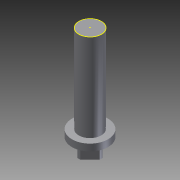
# Autodesk Inventor part: Поз12 Стержень
Saved by Autodesk Inventor 2012 SP2 (Build 160219200, 219)
## iProperties
Created: 2014-04-06
Part Number: Поз12 Стержень
Material: Default
Document SubType Name: Modeling
Designer: N750
Density: 1 g/cm^3
Author: N750
Autodesk Inventor part; units mm, degrees
ref_plane "YZ Plane" through (0, 0, 0) normal (1, 0, 0) x (0, 1, 0)
ref_plane "XZ Plane" through (0, 0, 0) normal (0, 1, 0) x (-1, 0, 0)
ref_plane "XY Plane" through (0, 0, 0) normal (0, 0, 1) x (1, 0, 0)
sketch "Эскиз1" plane through (0, 0, 0) normal (0, 0, 1) x (1, 0, 0)
  circle A0 centre (0, 0) radius 5
  dimension "d0" = 10
  constraints: 1 centre point, 1 coincident
  measures "d0" diameter of A0
extrude "Выдавливание1" add sketch "Эскиз1" along normal blind 6
sketch "Эскиз2" plane through (0, 0, 6) normal (0, 0, 1) x (1, 0, 0)
  circle A0 centre (0, 0) radius 5 projected
  line L0 (0, 5.6569) -> (5.6569, 0)
  line L1 (5.6569, 0) -> (0, -5.6569)
  line L2 (0, -5.6569) -> (-5.6569, 0)
  line L3 (-5.6569, 0) -> (0, 5.6569)
  dimension "d3" = 8
  constraints: 8 end point, 1 coincident, 9 other
  measures "d3" distance of L0.end L1.end
extrude "Выдавливание2" cut sketch "Эскиз2" against normal blind 6 contours A0 L1 L2 L3 L0 | A0 L0 L1 | A0 L3 L0 | L1 L2 A0 | A0 L2 L3 keep common part
sketch "Эскиз3" plane through (0, 0, 6) normal (0, 0, 1) x (1, 0, 0)
  line L0 (-0.7071, -4.9497) -> (-4.9497, -0.7071) projected
  arc A0 (-0.7071, -4.9497) -> (0.7071, -4.9497) centre (0, 0) ccw projected
  line L1 (4.9497, -0.7071) -> (0.7071, -4.9497) projected
  arc A1 (4.9497, -0.7071) -> (4.9497, 0.7071) centre (0, 0) ccw projected
  line L2 (0.7071, 4.9497) -> (4.9497, 0.7071) projected
  arc A2 (0.7071, 4.9497) -> (-0.7071, 4.9497) centre (0, 0) ccw projected
  line L3 (-4.9497, 0.7071) -> (-0.7071, 4.9497) projected
  arc A3 (-4.9497, 0.7071) -> (-4.9497, -0.7071) centre (0, 0) ccw projected
  circle A4 centre (0, 0) radius 8
  dimension "d6" = 16
  constraints: 1 centre point, 1 coincident
  measures "d6" diameter of A4
extrude "Выдавливание3" add sketch "Эскиз3" along normal blind 3
sketch "Эскиз4" plane through (0, 0, 9) normal (0, 0, 1) x (1, 0, 0)
  arc A0 (-4.9497, 0.7071) -> (-4.9497, -0.7071) centre (0, 0) ccw projected
  line L0 (-4.9497, 0.7071) -> (-0.7071, 4.9497) projected
  arc A1 (0.7071, 4.9497) -> (-0.7071, 4.9497) centre (0, 0) ccw projected
  line L1 (0.7071, 4.9497) -> (4.9497, 0.7071) projected
  arc A2 (4.9497, -0.7071) -> (4.9497, 0.7071) centre (0, 0) ccw projected
  line L2 (4.9497, -0.7071) -> (0.7071, -4.9497) projected
  arc A3 (-0.7071, -4.9497) -> (0.7071, -4.9497) centre (0, 0) ccw projected
  line L3 (-0.7071, -4.9497) -> (-4.9497, -0.7071) projected
extrude "Выдавливание4" add sketch "Эскиз4" against normal blind 3
sketch "Эскиз5" plane through (0, 0, 9) normal (0, 0, 1) x (1, 0, 0)
  circle A0 centre (0, 0) radius 8 projected
  circle A1 centre (0, 0) radius 5
  dimension "d11" = 10
  constraints: 1 centre point, 1 coincident
  measures "d11" diameter of A1
extrude "Выдавливание5" add sketch "Эскиз5" along normal blind 39 contours A1
sketch "Эскиз6" plane through (0, 0, 48) normal (0, 0, 1) x (1, 0, 0)
  circle A0 centre (0, 0) radius 5 projected
sketch "Эскиз7" plane through (0, 0, 48) normal (0, 0, 1) x (1, 0, 0)
  circle A0 centre (0, 0) radius 5 projected
